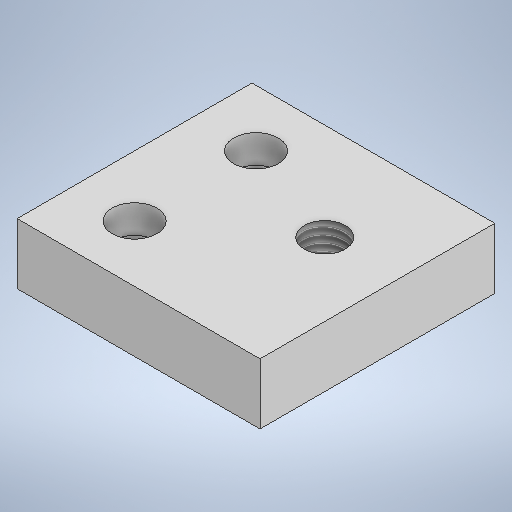
# Autodesk Inventor part: Lift Bracket other side
Saved by Autodesk Inventor 2026.2 (Build 302298010, 298A)
## iProperties
Created: 2026-04-27
Part Number: Lift Bracket other side
Material: Generic
Document SubType Name: Modeling
Designer: chanh
Density: 1 g/cm^3
Appearance: Default
Author: chanh
Autodesk Inventor part; units mm, degrees
ref_plane "YZ Plane" through (0, 0, 0) normal (1, 0, 0) x (0, 1, 0)
ref_plane "XZ Plane" through (0, 0, 0) normal (0, 1, 0) x (-1, 0, 0)
ref_plane "XY Plane" through (0, 0, 0) normal (0, 0, 1) x (1, 0, 0)
sketch "Sketch1" plane through (0, 0, 0) normal (0, 1, 0) x (-1, 0, 0)
  line L0 (30, 29) -> (-30, 29)
  line L1 (-30, 29) -> (-30, -29)
  line L2 (-30, -29) -> (30, -29)
  line L3 (30, -29) -> (30, 29)
  line L4 (30, 29) -> (-30, -29) construction
  line L5 (-30, 29) -> (30, -29) construction
  point P0 (0, 0)
  dimension "d0" = 60
  dimension "d1" = 58
  constraints: 12 end point, 2 midpoint, 2 parallel, 1 horizontal, 1 perpendicular
  measures "d0" distance of L1.end L2.end
  measures "d1" distance between parallel lines of L2 L0
extrude "Extrusion1" add sketch "Sketch1" along normal blind 15
sketch "Sketch2" plane through (0, 15, 0) normal (0, 1, 0) x (1, 0, 0)
  line L0 (30, -29) -> (30, 29) projected
  line L1 (30, 29) -> (-30, 29) projected
  line L2 (-30, 29) -> (-30, -29) projected
  line L3 (-30, -29) -> (30, -29) projected
  line L4 (-30, 0) -> (30, 0) construction
  point P0 (0, 0)
  point P1 (-15, -15)
  point P2 (-15, 15)
  point P3 (0, 0)
  point P4 (12, 5)
  dimension "d4" = 30
  dimension "d5" = 15
  dimension "d22" = 12
  dimension "d24" = 5
  constraints: 3 midpoint, 2 end point, 1 symmetric about line
  measures "d4" distance of point (-15, -15) point (-15, 15)
  measures "d5" horizontal distance of point (0, 0) point (-15, 15)
  measures "d22" horizontal distance of point (0, 0) point (12, 5)
  measures "d24" vertical distance of point (12, 5) point (0, 0)
hole "Hole1" at (12, 15, -5) direction (0, -1, 0) diameter 10.106 end through all thread size "M12x1.75" class "6H" standard "ISO Metric profile"
hole "Hole2" at (-15, 15, 15) at (-15, 15, -15) direction (0, -1, 0) diameter 6 end through all counterbore diameter 11 counterbore depth 7
body "Solid1"
